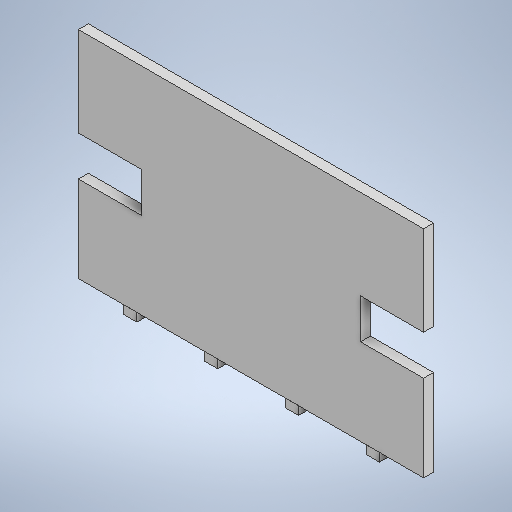
# Autodesk Inventor part: carcasa_piezaFrontal
Saved by Autodesk Inventor 2025.3 (Build 293356030, 356C)
## iProperties
Created: 2025-09-08
Part Number: carcasa_piezaFrontal
Material: Generic
Document SubType Name: Modeling
Designer: brene
Density: 1 g/cm^3
Appearance: Default
Author: brene
Autodesk Inventor part; units mm, degrees
ref_plane "YZ Plane" through (0, 0, 0) normal (1, 0, 0) x (0, 1, 0)
ref_plane "XZ Plane" through (0, 0, 0) normal (0, 1, 0) x (-1, 0, 0)
ref_plane "XY Plane" through (0, 0, 0) normal (0, 0, 1) x (1, 0, 0)
sketch "Sketch1" plane through (0, 0, 0) normal (0, 0, 1) x (1, 0, 0)
  line L0 (0, 0) -> (104, 0)
  line L1 (104, 0) -> (104, 65)
  line L2 (104, 65) -> (0, 65)
  line L3 (0, 65) -> (0, 0)
  dimension "d0" = 104
  dimension "d1" = 65
  constraints: 8 end point, 2 perpendicular, 1 horizontal, 1 parallel
  measures "d0" distance of L0.start L0.end
  measures "d1" distance of L0.end L1.end
extrude "Extrusion1" add sketch "Sketch1" along normal blind 3
sketch "Sketch2" plane through (0, 0, 3) normal (0, 0, 1) x (1, 0, 0)
  line L0 (0, 0) -> (104, 0) projected
  line L1 (52, 0) -> (52, 65)
  line L2 (104, 0) -> (104, 26)
  line L3 (104, 0) -> (104, 65) projected
  line L4 (104, 26) -> (85, 26)
  line L5 (85, 26) -> (85, 38)
  line L6 (85, 38) -> (104, 38)
  line L7 (0, 0) -> (0, 26)
  line L8 (0, 26) -> (19, 26)
  line L9 (19, 26) -> (19, 38)
  line L10 (19, 38) -> (0, 38)
  line L11 (0, 26) -> (0, 38)
  line L12 (0, 65) -> (0, 0) projected
  dimension "d8" = 26
  dimension "d9" = 19
  dimension "d10" = 12
  dimension "d11" = 19
  constraints: 20 end point, 4 symmetric about line, 2 perpendicular, 2 point on line, 1 collinear, 1 midpoint, 1 vertical
  measures "d8" distance of L0.end L2.end
  measures "d9" distance of L2.end L4.end
  measures "d10" distance of L4.end L5.end
  measures "d11" distance of L5.end L6.end
extrude "Extrusion2" cut sketch "Sketch2" against normal blind 50.975
sketch "Sketch3" plane through (0, 0, 0) normal (0, -1, 0) x (1, 0, 0)
  line L0 (0, 0) -> (0, 3) projected
  line L1 (0, 1.5) -> (104, 1.5)
  line L2 (104, 0) -> (104, 3) projected
  line L3 (0, 3) -> (104, 3) projected
  line L4 (52, 3) -> (52, 0)
  line L5 (0, 0) -> (104, 0) projected
  line L6 (52, 1.5) -> (41.8165, 1.5)
  line L7 (52, 1.5) -> (62.1835, 1.5)
  line L8 (41.8165, 1.5) -> (37.8165, 1.5)
  line L9 (39.8165, 1.5) -> (37.8165, 1.5)
  line L10 (37.8165, 1.5) -> (37.8165, 2.85)
  line L11 (41.8165, 1.5) -> (41.8165, 0.15)
  line L12 (37.8165, 2.85) -> (41.8165, 2.85)
  line L13 (41.8165, 2.85) -> (41.8165, 0.15)
  line L14 (41.8165, 0.15) -> (37.8165, 0.15)
  line L15 (37.8165, 0.15) -> (37.8165, 2.85)
  line L16 (66.1835, 1.5) -> (66.1835, 2.85)
  line L17 (66.1835, 2.85) -> (62.1835, 2.85)
  line L18 (62.1835, 2.85) -> (62.1835, 0.15)
  line L19 (62.1835, 0.15) -> (66.1835, 0.15)
  line L20 (66.1835, 0.15) -> (66.1835, 2.85)
  line L21 (37.8165, 1.5) -> (17.4495, 1.5)
  line L22 (27.633, 1.5) -> (27.633, 3)
  line L23 (17.4495, 2.85) -> (13.4495, 2.85)
  line L24 (13.4495, 2.85) -> (13.4495, 0.15)
  line L25 (13.4495, 0.15) -> (17.4495, 0.15)
  line L26 (17.4495, 0.15) -> (17.4495, 2.85)
  line L27 (86.5505, 0.15) -> (86.5505, 2.85)
  line L28 (86.5505, 2.85) -> (90.5505, 2.85)
  line L29 (90.5505, 2.85) -> (90.5505, 0.15)
  line L30 (90.5505, 0.15) -> (86.5505, 0.15)
  dimension "d14" = 10.1835
  dimension "d15" = 10.1835
  dimension "d16" = 4
  dimension "d17" = 2
  dimension "d18" = 1.35
  dimension "d19" = 1.35
  dimension "d20" = 20.367
  constraints: 54 end point, 13 symmetric about line, 7 midpoint, 5 point on line, 3 perpendicular, 2 parallel, 1 collinear, 1 horizontal, 1 vertical
  measures "d14" distance of L6.start L6.end
  measures "d15" distance of L6.start L7.end
  measures "d16" distance of L6.end L8.end
  measures "d17" distance of L9.start L8.end
  measures "d18" distance of L8.end L10.end
  measures "d19" distance of L6.end L11.end
  measures "d20" distance of L8.end L21.end
extrude "Extrusion3" add sketch "Sketch3" along normal blind 2.7 contours L24 L23 L26 L1 | L1 L26 L25 L24 | L11 L14 L15 L1 | L1 L10 L12 L13 | L18 L17 L16 L1 | L1 L20 L19 L18 | L29 L30 L27 L1 | L1 L27 L28 L29
body "Solid1"
